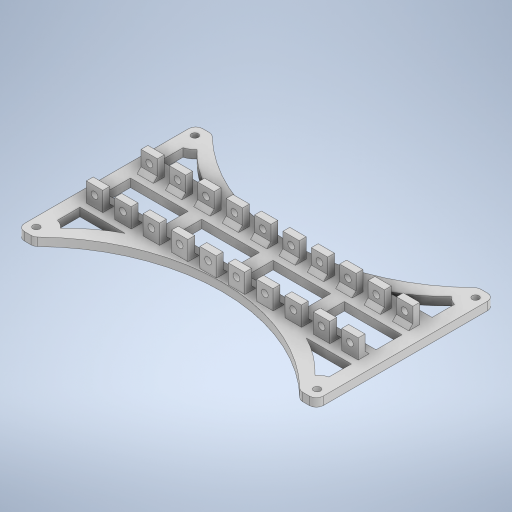
# Autodesk Inventor part: m500 mount
Saved by Autodesk Inventor 2023 (Build 270158000, 158)
## iProperties
Created: 2022-08-10
Part Number: m500 mount
Material: Generic
Document SubType Name: Modeling
Designer: Eli
Density: 1 g/cm^3
Appearance: Default
Author: Eli
Autodesk Inventor part; units mm, degrees
ref_plane "YZ Plane" through (0, 0, 0) normal (1, 0, 0) x (0, 1, 0)
sketch "Sketch1" plane through (0, 0, 0) normal (0, 1, 0) x (-1, 0, 0)
  line L0 (0, 0) -> (-138.43, 0)
  line L1 (-138.43, 0) -> (-138.43, -82.55)
  line L2 (-138.43, -82.55) -> (0, -82.55)
  line L3 (0, -82.55) -> (0, 0)
  circle A0 centre (-4.191, -4.572) radius 1.5875
  circle A1 centre (-4.191, -77.978) radius 1.5875
  line L4 (0, -41.275) -> (-138.43, -41.275) construction
  circle A2 centre (-134.239, -4.572) radius 1.5875
  line L5 (-69.215, 0) -> (-69.215, -82.55) construction
  circle A3 centre (-134.239, -77.978) radius 1.5875
  line L6 (-81.28, -82.55) -> (-113.03, -82.55)
  arc A4 (-7.62, -82.55) -> (-130.81, -82.55) centre (-69.215, -144.145) ccw
  arc A5 (-130.81, 0) -> (-7.62, 0) centre (-69.215, 61.595) ccw
  point P0 (-130.81, -82.55)
  point P1 (-7.62, 0)
  point P2 (-130.81, 0)
  dimension "d0" = 82.55
  dimension "d1" = 138.43
  dimension "d2" = 73.406
  dimension "d3" = 3.175
  dimension "d4" = 130.048
  dimension "d39" = 7.62
  dimension "d40" = 7.62
  dimension "d41" = 0
  dimension "d42" = 90
  constraints: 14 end point, 6 centre point, 6 symmetric about line, 4 midpoint, 4 point on circle, 3 equal radius, 2 horizontal, 2 parallel, 2 point on line, 1 perpendicular, 1 other
  measures "d0" distance of L2.end L0.start
  measures "d1" distance of L1.end L2.end
  measures "d2" distance of A1.centre A0.centre
  measures "d3" diameter of A0
  measures "d4" distance of A0.centre A2.centre
  measures "d39" distance from line of L3 A4.start
  measures "d40" distance from line of L1 A4.end
  measures "d41" distance from line of L2 A4.end
ref_plane "Work Plane2" through (0, 3.81, 0) normal (0, 1, 0) x (1, 0, 0)
sketch "Sketch2" plane through (0, 3.81, 0) normal (0, 1, 0) x (1, 0, 0)
  line L0 (124.46, 54.2544) -> (132.08, 54.2544)
  line L1 (132.08, 54.2544) -> (132.08, 51.0794)
  line L2 (132.08, 51.0794) -> (124.46, 51.0794)
  line L3 (124.46, 51.0794) -> (124.46, 54.2544)
  line L4 (138.43, 0) -> (138.43, 80.01) projected
  line L5 (124.46, 28.9306) -> (132.08, 28.9306)
  line L6 (132.08, 28.9306) -> (132.08, 25.7556)
  line L7 (132.08, 25.7556) -> (124.46, 25.7556)
  line L8 (124.46, 25.7556) -> (124.46, 28.9306)
  line L9 (138.43, 0) -> (138.43, 80.01) construction
  line L10 (138.43, 40.005) -> (0, 40.005) construction
  line L11 (0, 80.01) -> (0, 0) construction
  point P0 (138.43, 3.175)
  point P1 (138.43, 76.835)
  point P2 (0, 76.835)
  point P3 (0, 3.175)
  dimension "d13" = 6.35
  dimension "d14" = 7.62
  dimension "d15" = 3.175
  dimension "d16" = 28.4988
  constraints: 18 end point, 4 parallel, 2 equal length, 2 horizontal, 2 midpoint, 2 perpendicular, 1 collinear, 1 other
  measures "d13" distance between parallel lines of L4 L1
  measures "d14" distance of L0.start L0.end
  measures "d15" distance of L0.end L1.end
  measures "d16" distance between parallel lines of L7 L0
extrude "Extrusion2" add sketch "Sketch2" along normal blind 8.89
ref_plane "Work Plane3" through (124.46, 3.81, -25.7556) normal (0, 0, 1) x (1, 0, 0)
sketch "Sketch3" plane through (124.46, 3.81, -25.7556) normal (0, 0, 1) x (1, 0, 0)
  line L0 (7.62, 0) -> (7.62, 8.89) projected
  line L1 (-124.46, 0) -> (13.97, 0) projected
  point P0 (-124.46, -3.81)
  point P1 (3.81, 5.08)
  point P2 (3.752, 0)
  point P3 (10.795, 0)
  point P4 (-121.285, 0)
  dimension "d27" = 3.81
  dimension "d28" = 5.08
  measures "d27" distance from line of L0 point (3.81, 5.08)
  measures "d28" distance from line of L1 point (3.81, 5.08)
hole "Hole1" at (128.27, 8.89, -25.7556) direction (0, 0, -1) diameter 3.175 depth 28.4988
extrude "Extrusion3" add sketch "Sketch1" along normal blind 3.81 contours L3 L2 A4 L1 L0 A5
pattern_linear "Rectangular Pattern2" count 10 spacing 13.1445 along (-1, 0, 0) of "Extrusion2", "Hole1"
fillet "Fillet2" radius 3.175 8 edges at (0, 1.905, 0) (7.62, 1.905, 0) (130.81, 1.905, 0) (138.43, 1.905, 0) (138.43, 1.905, -82.55) (130.81, 1.905, -82.55) (7.62, 1.905, -82.55) (0, 1.905, -82.55)
chamfer "Chamfer1" distance 1.905 angle 45 20 edges at (128.27, 3.81, -51.0794) (128.27, 3.81, -28.9306) (115.1255, 3.81, -28.9306) (101.981, 3.81, -28.9306) (88.8365, 3.81, -28.9306) (75.692, 3.81, -28.9306) (62.5475, 3.81, -28.9306) (49.403, 3.81, -28.9306) (36.2585, 3.81, -28.9306) (23.114, 3.81, -28.9306) (9.9695, 3.81, -28.9306) (115.1255, 3.81, -51.0794) (101.981, 3.81, -51.0794) (88.8365, 3.81, -51.0794) (75.692, 3.81, -51.0794) (62.5475, 3.81, -51.0794) (49.403, 3.81, -51.0794) (36.2585, 3.81, -51.0794) (23.114, 3.81, -51.0794) (9.9695, 3.81, -51.0794)
sketch "Sketch5" plane through (0, 3.81, 0) normal (0, 1, 0) x (1, 0, 0)
  line L0 (6.35, 5.08) -> (6.35, 22.5806)
  line L1 (6.35, 22.5806) -> (27.2203, 22.5806)
  arc A0 (27.2203, 22.5806) -> (6.35, 5.08) centre (57.8461, -35.1368) ccw
  line L2 (0, 79.375) -> (0, 3.175) projected
  line L3 (3.175, 0) -> (6.3186, 0) projected
  line L4 (6.1595, 25.7556) -> (13.7795, 25.7556) projected
  circle A1 centre (4.191, 4.572) radius 7.9375
  circle A2 centre (4.191, 4.572) radius 1.5875 projected
  line L5 (0, 79.375) -> (0, 3.175) construction
  line L6 (0, 41.275) -> (138.43, 41.275) construction
  line L7 (138.43, 3.175) -> (138.43, 79.375) construction
  line L8 (69.215, 41.275) -> (69.215, 57.0365) construction
  arc A3 (8.5305, 81.6528) -> (129.8995, 81.6528) centre (69.215, 144.145) ccw construction
  line L9 (132.08, 5.08) -> (132.08, 22.5806)
  line L10 (132.08, 22.5806) -> (111.2097, 22.5806)
  arc A4 (132.08, 5.08) -> (111.2097, 22.5806) centre (80.5839, -35.1368) ccw
  circle A5 centre (134.239, 4.572) radius 7.9375
  line L11 (6.35, 77.47) -> (6.35, 59.9694)
  line L12 (6.35, 59.9694) -> (27.2203, 59.9694)
  arc A6 (6.35, 77.47) -> (27.2203, 59.9694) centre (57.8461, 117.6868) ccw
  circle A7 centre (4.191, 77.978) radius 7.9375
  circle A8 centre (134.239, 77.978) radius 7.9375
  line L13 (132.08, 77.47) -> (132.08, 59.9694)
  line L14 (132.08, 59.9694) -> (111.2097, 59.9694)
  arc A9 (111.2097, 59.9694) -> (132.08, 77.47) centre (80.5839, 117.6868) ccw
  line L15 (6.35, 45.9994) -> (132.08, 45.9994)
  line L16 (132.08, 45.9994) -> (132.08, 34.0106)
  line L17 (132.08, 34.0106) -> (6.35, 34.0106)
  line L18 (6.35, 34.0106) -> (6.35, 45.9994)
  line L19 (6.1595, 49.1744) -> (13.7795, 49.1744) projected
  line L20 (26.924, 30.8356) -> (19.304, 30.8356) projected
  line L21 (66.04, 45.9994) -> (72.39, 45.9994)
  line L22 (72.39, 45.9994) -> (72.39, 34.0106)
  line L23 (72.39, 34.0106) -> (66.04, 34.0106)
  line L24 (66.04, 34.0106) -> (66.04, 45.9994)
  line L25 (33.02, 45.9994) -> (39.37, 45.9994)
  line L26 (39.37, 45.9994) -> (39.37, 34.0106)
  line L27 (39.37, 34.0106) -> (33.02, 34.0106)
  line L28 (33.02, 34.0106) -> (33.02, 45.9994)
  line L29 (66.04, 40.005) -> (39.37, 40.005) construction
  line L30 (33.02, 40.005) -> (6.35, 40.005) construction
  line L31 (99.06, 45.9994) -> (99.06, 34.0106)
  line L32 (105.41, 34.0106) -> (105.41, 45.9994)
  point P0 (0, 0)
  point P1 (128.148, 9.6616)
  point P2 (132.08, 12.2102)
  point P3 (132.08, 70.3398)
  point P4 (128.148, 72.8884)
  point P5 (10.282, 72.8884)
  point P6 (6.35, 70.3398)
  point P7 (6.35, 12.2102)
  point P8 (10.282, 9.6616)
  dimension "d54" = 6.35
  dimension "d55" = 5.08
  dimension "d56" = 3.175
  dimension "d57" = 6.35
  dimension "d58" = 6.35
  dimension "d59" = 6.35
  dimension "d60" = 3.175
  dimension "d61" = 3.175
  dimension "d64" = 6.35
  dimension "d65" = 6.35
  constraints: 52 end point, 19 symmetric about line, 9 point on circle, 8 centre point, 7 midpoint, 6 parallel, 5 perpendicular, 4 point on line, 3 horizontal, 1 coincident, 1 collinear, 1 vertical, 7 other
  measures "d54" distance between parallel lines of L2 L0
  measures "d55" distance from line of L3 L0.start
  measures "d56" distance between parallel lines of L4 L1
  measures "d57" radial gap between concentric circles of A1 A2
  measures "d58" distance between parallel lines of L2 L18
  measures "d59" distance between parallel lines of L7 L16
  measures "d60" distance between parallel lines of L19 L15
  measures "d61" distance between parallel lines of L20 L17
  measures "d64" distance between parallel lines of L22 L24
  measures "d65" distance between parallel lines of L26 L28
extrude "Extrusion5" cut sketch "Sketch5" against normal blind 25.4 contours L0 L1 A0 A1 | A5 A4 L10 L9 | A7 A6 L12 L11 | A8 L13 L14 A9 | L15 L28 L17 L18 | L15 L24 L17 L26 | L15 L31 L17 L22 | L15 L16 L17 L32
body "Solid1"
